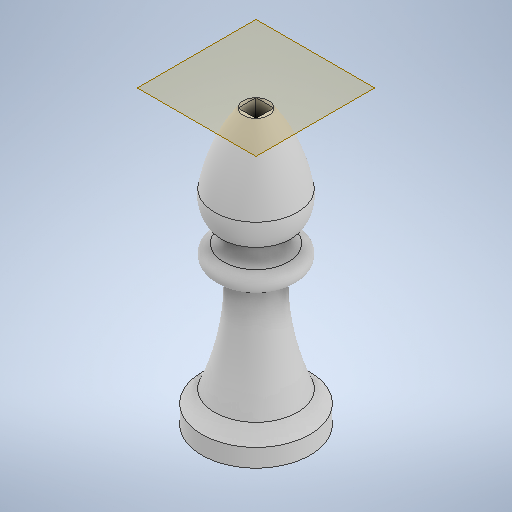
# Autodesk Inventor part: PawnUntagged
Saved by Autodesk Inventor 2025.2 (Build 292293000, 293)
## iProperties
Created: 2025-02-26
Part Number: PawnUntagged
Material: Generic
Document SubType Name: Modeling
Designer: Marcu
Density: 1 g/cm^3
Appearance: Default
Author: Marcu
Autodesk Inventor part; units mm, degrees
ref_plane "YZ Plane" through (0, 0, 0) normal (1, 0, 0) x (0, 1, 0)
ref_plane "XY Plane" through (0, 0, 0) normal (0, 0, 1) x (1, 0, 0)
sketch "Sketch1" plane through (0, 0, 0) normal (1, 0, 0) x (0, 1, 0)
  line L0 (4, 0.0001) -> (4, 2.5001)
  line L1 (4, 2.5001) -> (0, 2.5001)
  line L2 (0, 2.5001) -> (0, 15)
  line L3 (0, 15) -> (5, 15)
  line L4 (5, 15) -> (8.5355, 11.4645)
  line L5 (38.5355, 8.8749) -> (38.5355, 8.9645)
  line L6 (41.0355, 11.4645) -> (41.0355, 11.4645)
  line L7 (43.5355, 8.9645) -> (43.5355, 9.0096)
  line L8 (46.0356, 6.4646) -> (46.0012, 6.4646)
  arc A0 (43.5355, 8.9645) -> (41.0355, 11.4645) centre (41.0355, 8.9645) ccw
  arc A1 (41.0355, 11.4645) -> (38.5355, 8.9645) centre (41.0355, 8.9645) ccw
  arc A2 (8.5355, 11.4645) -> (36.0825, 6.3754) centre (34.7686, 76.363) ccw
  line L9 (4, 0.0001) -> (80.0002, 0.0001)
  line L10 (46.0356, 6.4646) -> (46.0012, 6.4646)
  line L11 (80.0002, 0.0001) -> (80.0002, 0.0001)
  line L12 (77.5002, 2.5001) -> (77.5002, 2.5001)
  arc A3 (77.5002, 2.5001) -> (56.7241, 11.4495) centre (49.6175, -33.6394) ccw
  arc A4 (43.5355, 8.9645) -> (48.4415, 8.2845) centre (46.0356, 8.9645) ccw
  arc A5 (56.7241, 11.4495) -> (49.3393, 9.5985) centre (55.209, 1.837) ccw
  line L13 (80.0002, 0.0001) -> (80.0002, 0.0001)
  line L14 (77.5002, 2.5001) -> (77.5002, 2.5001)
  arc A6 (80.0002, 0.0001) -> (77.5002, 2.5001) centre (77.5002, 0.0001) ccw
  arc A7 (49.3393, 9.5985) -> (48.4415, 8.2845) centre (50.8472, 7.6045) ccw
  arc A8 (36.0825, 6.3754) -> (38.5355, 8.8749) centre (36.0355, 8.8749) ccw
  point P0 (0, 0)
  point P1 (38.5355, 6.4645)
  point P2 (38.5355, 11.4645)
  point P3 (43.5355, 11.4645)
  point P4 (43.5355, 6.4646)
  point P5 (80.0002, 2.5001)
  point P6 (77.5002, 2.5001)
  dimension "d0" = 4
  dimension "d1" = 2.5
  dimension "d2" = 15
  dimension "d3" = 5
  dimension "d4" = 5
  dimension "d5" = 135
  dimension "d25" = 5
  dimension "d26" = 5
  dimension "d36" = 70
  dimension "d47" = 2.5
  dimension "d48" = 2.5
  dimension "d49" = 2.5
  dimension "d51" = 2.5
  constraints: 30 end point, 20 point on circle, 12 tangent, 9 centre point, 9 point on line, 4 horizontal, 4 perpendicular, 3 vertical, 1 equal radius
  measures "d0" distance of point (0, 0) L0.start
  measures "d1" distance of L0.start L0.end
  measures "d2" distance of point (0, 0) L2.end
  measures "d3" distance of L2.end L3.end
  measures "d4" distance of L3.end L4.end
  measures "d5" angle of L3 L4
  measures "d25" distance of point (38.536, 6.464) point (38.536, 11.464)
  measures "d26" distance of point (38.536, 11.464) point (43.536, 11.464)
  measures "d36" radius of A2
  measures "d47" distance of L11.end point (80, 2.5)
  measures "d48" distance of point (80, 2.5) L12.start
  measures "d49" radius of A6
  measures "d51" radius of A8
revolve "Revolution1" add sketch "Sketch1" angle 360 about axis through (0, 4, 0.0001) along (0, 1, 0)
ref_plane "Work Plane1" through (0, 80.9625, 0) normal (0, 1, 0) x (-1, 0, 0)
sketch "Sketch2" plane through (0, 80.9625, 0) normal (0, 1, 0) x (-1, 0, 0)
  line L0 (2.5, -2.5) -> (-2.5, -2.5)
  line L1 (-2.5, -2.5) -> (-2.5, 2.5)
  line L2 (-2.5, 2.5) -> (2.5, 2.5)
  line L3 (2.5, 2.5) -> (2.5, -2.5)
  point P0 (0, 0)
  dimension "d53" = 5
  dimension "d54" = 2.5
  dimension "d55" = 2.5
  dimension "d56" = 5
  constraints: 8 end point, 2 parallel, 1 horizontal, 1 perpendicular
  measures "d53" distance between parallel lines of L3 L1
  measures "d54" distance from line of point (0, 0) L1
  measures "d55" distance from line of point (0, 0) L2
  measures "d56" distance between parallel lines of L0 L2
extrude "Extrusion1" cut sketch "Sketch2" against normal blind 12
sketch "Sketch3" plane through (0, 80.9625, 0) normal (0, 1, 0) x (-1, 0, 0)
  circle A0 centre (0, 0.0001) radius 2.5 projected
  circle A1 centre (0, 0.0001) radius 3.5355
  point P0 (0, 0)
  constraints: 1 centre point, 1 coincident
extrude "Extrusion2" cut sketch "Sketch3" against normal blind 4.85 contours A0 | A1
body "Solid1"
